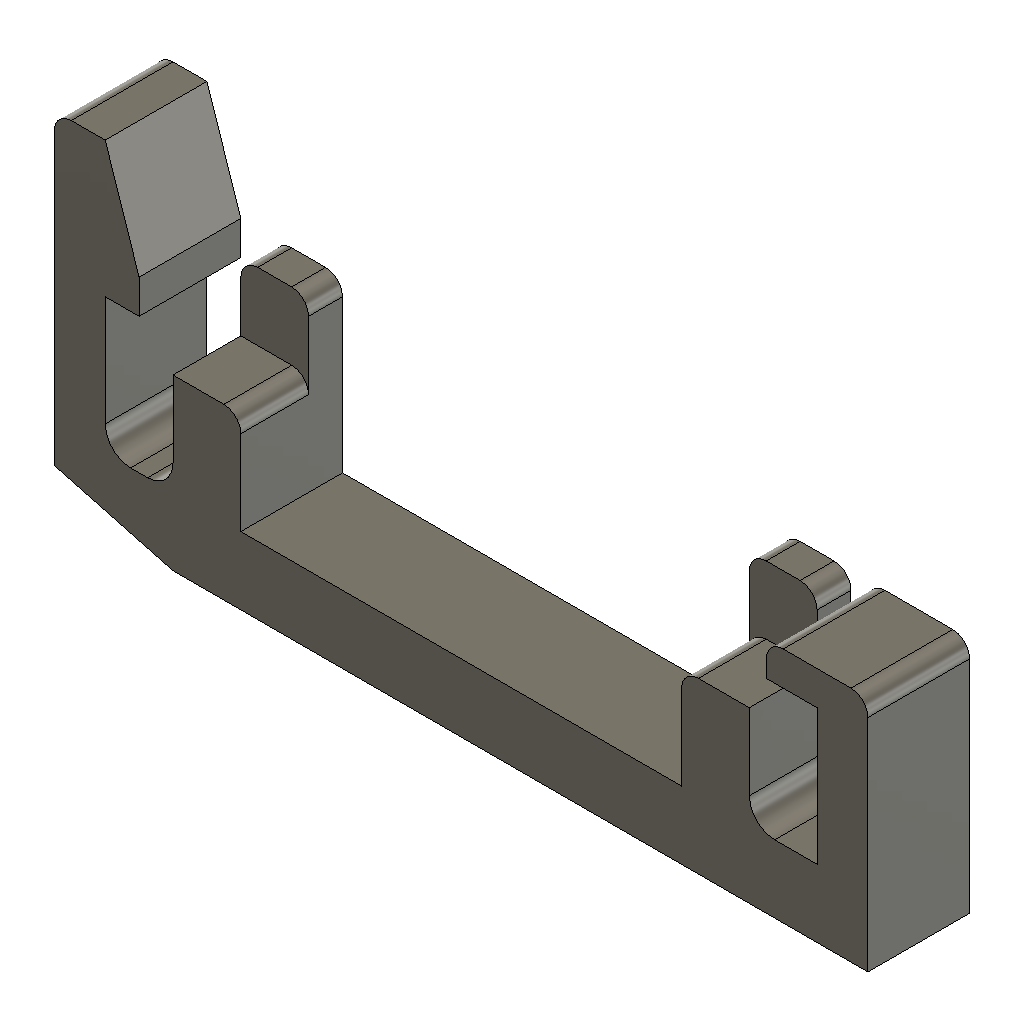
Clip (Autodesk Fusion 360 design; units mm, degrees)
Autodesk Fusion 360 part; units mm, degrees
sketch "Base" plane through (0, 0, 0) normal (0, 0, 1) x (1, 0, 0)
  line L0 (0, 0) -> (0, -9.0622)
  line L1 (24, -10) -> (24, -3)
  line L2 (22.5, -4) -> (22.5, -8)
  line L3 (20.5, -5) -> (3.5, -5)
  line L4 (1.5, -8) -> (1.5, -4)
  line L5 (1.5, 0) -> (0, 0)
  line L6 (3.5, -5) -> (3.5, -8)
  line L7 (3.5, -8) -> (1.5, -8)
  line L8 (22.5, -8) -> (20.5, -8)
  line L9 (20.5, -5) -> (20.5, -8)
  line L10 (24, -3) -> (21, -3)
  line L11 (21, -3) -> (21, -4)
  line L12 (21, -4) -> (22.5, -4)
  line L13 (1.5, 0) -> (2.5, -3)
  line L14 (2.5, -3) -> (2.5, -4)
  line L15 (2.5, -4) -> (1.5, -4)
  line L16 (21, -4) -> (2.5, -4) construction
  line L17 (3.5, -10) -> (0, -9.0622)
  line L18 (3.5, -8) -> (3.5, -10) construction
  line L19 (3.5, -10) -> (24, -10)
  dimension "d4" = 21
  dimension "d5" = 3.5
  dimension "d7" = 2
  dimension "d8" = 2
  dimension "d10" = 1
  dimension "d11" = 3
  dimension "d15" = 1
  dimension "d16" = 4
  dimension "d17" = 4
  dimension "d18" = 2.5
  dimension "d19" = 1.5
  dimension "d20" = 3
  dimension "d48" = 6
  dimension "d49" = 165
  dimension "d50" = 1.5
  constraint coincident L0.start L5.end
  constraint vertical L0
  constraint perpendicular L2 L3
  constraint perpendicular L3 L4
  constraint perpendicular L0 L5
  constraint perpendicular L3 L6
  constraint perpendicular L6 L7
  constraint coincident L4.start L7.end
  constraint perpendicular L2 L8
  constraint perpendicular L8 L9
  constraint coincident L2.end L8.start
  constraint perpendicular L2 L10
  constraint perpendicular L10 L11
  constraint perpendicular L2 L12
  constraint coincident L1.end L10.start
  constraint perpendicular L5 L14
  constraint perpendicular L4 L15
  constraint horizontal L16
  constraint vertical L18
  constraint perpendicular L1 L19
  measures "d4" distance of L2 L4
  measures "d5" distance of L0 L6
  measures "d7" distance of L2 L9
  measures "d8" distance of L4 L6
  measures "d10" distance of L10.end L11.end
  measures "d11" distance of L1.end L10.end
  measures "d15" distance of L13.end L14.end
  measures "d16" distance of L2.end L2.start
  measures "d17" distance of L4.start L4.end
  measures "d18" distance of L0 L14
  measures "d19" distance of L5.start L0.start
  measures "d20" distance of L5 L13.end
  measures "d48" distance of L16 L19
  measures "d49" angle of L17 L19
  measures "d50" distance of L1 L2
extrude "Extrude1" add sketch "Base" along normal blind 3
sketch "Cutout" plane through (0, -5, 0) normal (0, 1, 0) x (-1, 0, 0)
  line L0 (-20.5, 0) -> (-3.5, 0)
  line L1 (-3.5, 0) -> (-3.5, 3)
  line L2 (-3.5, 3) -> (-20.5, 3)
  line L3 (-20.5, 3) -> (-20.5, 0)
  line L4 (-5.5, 0) -> (-18.5, 0)
  line L5 (-18.5, 0) -> (-18.5, 3)
  line L6 (-18.5, 3) -> (-5.5, 3)
  line L7 (-5.5, 3) -> (-5.5, 0)
  dimension "d31" = 13
  constraint horizontal L4
  constraint vertical L5
  constraint horizontal L6
  constraint vertical L7
  constraint coincident L2 L5.end
  constraint coincident L0 L4.start
  constraint midpoint L0 L4
  measures "d31" distance of L5 L7
extrude "Extrude2" cut sketch "Cutout" against normal blind 3 contours L0 L2 L4 L5 L6 L7
sketch "Stand" plane through (0, -5, 0) normal (0, 1, 0) x (-1, 0, 0)
  line L0 (-5.5, 3) -> (-5.5, 0)
  line L1 (-5.5, 0) -> (-3.5, 0)
  line L2 (-3.5, 0) -> (-3.5, 3)
  line L3 (-3.5, 3) -> (-5.5, 3)
  line L4 (-3.5, 0) -> (-5.5, 0)
  line L5 (-5.5, 0) -> (-5.5, 1)
  line L6 (-5.5, 1) -> (-3.5, 1)
  line L7 (-3.5, 1) -> (-3.5, 0)
  dimension "d32" = 1
  constraint horizontal L4
  constraint vertical L5
  constraint horizontal L6
  constraint vertical L7
  constraint coincident L0 L5.end
  constraint coincident L1.end L2.start
  measures "d32" distance of L0.end L5.end
sketch "Stand (1)" plane through (0, -5, 0) normal (0, 1, 0) x (-1, 0, 0)
  line L0 (-18.5, 0) -> (-18.5, 3)
  line L1 (-18.5, 3) -> (-20.5, 3)
  line L2 (-20.5, 3) -> (-20.5, 0)
  line L3 (-20.5, 0) -> (-18.5, 0)
  line L4 (-18.5, 0) -> (-20.5, 0)
  line L5 (-20.5, 0) -> (-20.5, 1)
  line L6 (-20.5, 1) -> (-18.5, 1)
  line L7 (-18.5, 1) -> (-18.5, 0)
  dimension "d33" = 1
  constraint horizontal L4
  constraint vertical L5
  constraint horizontal L6
  constraint vertical L7
  constraint coincident L2 L5.end
  constraint coincident L0.start L3.end
  measures "d33" distance of L0.start L6.end
extrude "Extrude3" add sketch "Stand" sketch "Stand (1)" along normal blind 2 contours L0 L1 L2 L4 L5 L6 L7 of sketch 2 contours L0 L2 L3 L4 L5 L6 L7
fillet "Fillet1" radius 0.5 9 edges at (5.5, -3, 0.5) (5.5, -5, 2) (18.5, -5, 2) (18.5, -3, 0.5) (20.5, -3, 0.5) (3.5, -3, 0.5) (0, 0, 1.5) (24, -3, 1.5) (21, -3, 1.5)
fillet "Fillet1" radius 0.75 3 edges at (1.5, -8, 1.5) (20.5, -8, 1.5) (3.5, -8, 1.5)
equation "CLIP_PCB_SIZE = 21 mm"
equation "d4 = CLIP_PCB_SIZE"
equation "d31 = CLIP_PCB_SIZE - 8 mm"
named bodies: "PCB Clip"
